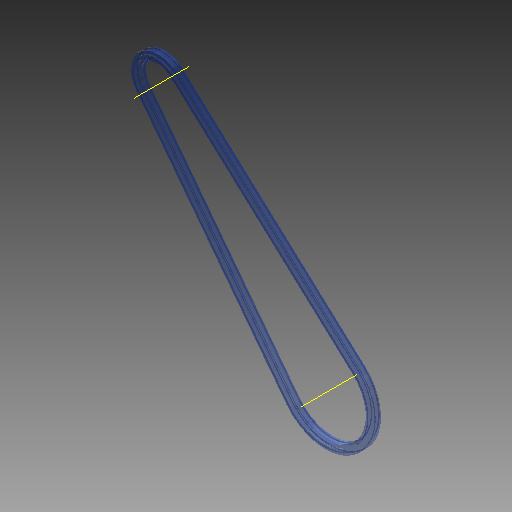
# Autodesk Inventor part: Roller Chain
Saved by Autodesk Inventor 2019.4 (Build 234330000, 330)
## iProperties
Created: 2020-01-22
Part Number: Roller Chain
Material: Generic
Document SubType Name: Modeling
Designer: admin
Mass: 22.4217 g
Surface Area: 188.754 cm^2
Volume: 22.4217 cm^3
Density: 1 g/cm^3
Appearance: Clear - Blue
CustomPartVersion: 1
Author: admin
Autodesk Inventor part; units mm, degrees
ref_plane "YZ Plane" through (0, 0, 0) normal (1, 0, 0) x (0, 1, 0)
ref_plane "XZ Plane" through (0, 0, 0) normal (0, 1, 0) x (-1, 0, 0)
ref_plane "XY Plane" through (0, 0, 0) normal (0, 0, 1) x (1, 0, 0)
ref_plane "Work Plane2" through (-37.1709, 52.6893, 0) normal (-1, 0, 0) x (0, 0, 1)
ref_plane "Work Plane3" through (-181.1709, 209.8263, 0) normal (0.5807817, -0.8140594, 0) x (0, 0, 1)
sketch "Path" plane through (0, 0, 0) normal (0, 0, 1) x (1, 0, 0)
  arc A0 (-67.5789, 29.4573) -> (-11.3791, 80.9586) centre (-37.1709, 52.6893) ccw
  arc A1 (-168.204, 224.0388) -> (-196.4586, 198.1463) centre (-181.1709, 209.8263) ccw
  line L0 (-168.204, 224.0388) -> (-11.3791, 80.9586)
  line L1 (-67.5789, 29.4573) -> (-196.4586, 198.1463)
  dimension "d31" = 7.11
  constraints: 4 end point, 4 point on circle, 2 centre point
ref_plane "Section Plane" through (-11.3791, 80.9586, 0) normal (-0.7387381, 0.6739926, 0) x (0, 0, 1)
sketch "Section Sketch" plane through (-11.3791, 80.9586, 0) normal (-0.7387381, 0.6739926, 0) x (0, 0, 1)
  line L0 (-4.3, -1.155) -> (4.3, -1.155)
  line L1 (4.3, -1.155) -> (4.3, 1.155)
  line L2 (4.3, 1.155) -> (-4.3, 1.155)
  line L3 (-4.3, 1.155) -> (-4.3, -1.155)
  line L4 (-1.5, -2.5) -> (1.5, -2.5)
  line L5 (1.5, -2.5) -> (1.5, 2.5)
  line L6 (1.5, 2.5) -> (-1.5, 2.5)
  line L7 (-1.5, 2.5) -> (-1.5, -2.5)
  line L8 (-1.5, 0) -> (1.5, 0) construction
  line L9 (-3, -3.555) -> (-1.5, -3.555)
  line L10 (-1.5, -3.555) -> (-1.5, 3.555)
  line L11 (-1.5, 3.555) -> (-3, 3.555)
  line L12 (-3, 3.555) -> (-3, -3.555)
  line L13 (1.5, -3.555) -> (3, -3.555)
  line L14 (3, -3.555) -> (3, 3.555)
  line L15 (3, 3.555) -> (1.5, 3.555)
  line L16 (1.5, 3.555) -> (1.5, -3.555)
  line L17 (-4.3, 0) -> (4.3, 0) construction
  point P0 (0, 0)
  point P1 (0, 0)
  dimension "d21" = 2.31
  dimension "d22" = 5
  dimension "d23" = 3
  dimension "d24" = 1.5
  dimension "d31" = 7.11
  dimension "d32" = 8.6
  constraints: 36 end point, 8 midpoint, 8 parallel, 4 horizontal, 4 perpendicular, 3 collinear, 1 coincident, 1 other
  measures "d21" distance between parallel lines of L2 L0
  measures "d22" distance between parallel lines of L6 L4
  measures "d23" distance between parallel lines of L5 L7
  measures "d24" distance between parallel lines of L12 L10
  measures "d31" distance between parallel lines of L11 L9
  measures "d32" distance between parallel lines of L1 L3
sweep "Solid" add profiles "Section Sketch" path "Path" path curves L1 A1 L0 A0
pattern_of_one "Strand Pattern"
equation "\"d21\" = da_d2"
equation "\"d22\" = da_d1"
equation "\"d23\" = da_b1"
equation "\"d24\" = da_t1 + da_t2"
equation "\"d30\" = da_pt"
equation "\"da_p\" = 8"
equation "\"da_b1\" = 3"
equation "\"da_h2\" = 7.11"
equation "\"da_h3\" = 7.11"
equation "\"da_d1\" = 5"
equation "\"da_d2\" = 2.31"
equation "\"da_pt\" = 5.64"
equation "\"da_b\" = 8.6"
equation "\"da_t1\" = 0.75"
equation "\"da_t2\" = 0.75"
body "Solid1"
